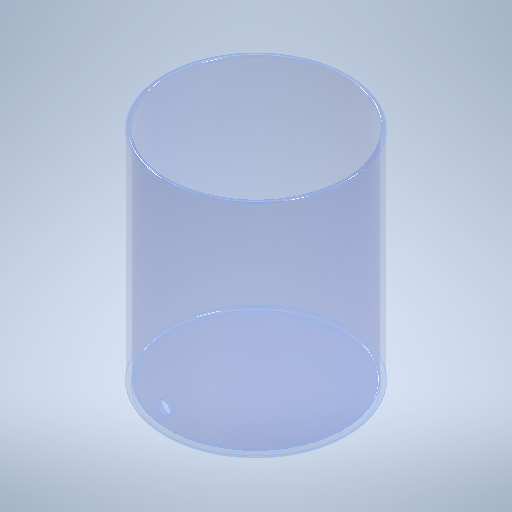
# Autodesk Inventor part: Reservoir
Saved by Autodesk Inventor 2025.2 (Build 292293000, 293)
## iProperties
Created: 2025-05-29
Part Number: Reservoir
Material: Generic
Document SubType Name: Modeling
Designer: Simon
Density: 1 g/cm^3
Appearance: Tropical Blue
Author: Simon
Autodesk Inventor part; units mm, degrees
ref_plane "YZ Plane" through (0, 0, 0) normal (1, 0, 0) x (0, 1, 0)
ref_plane "XZ Plane" through (0, 0, 0) normal (0, 1, 0) x (-1, 0, 0)
ref_plane "XY Plane" through (0, 0, 0) normal (0, 0, 1) x (1, 0, 0)
sketch "Sketch1" plane through (0, 0, 0) normal (0, 1, 0) x (-1, 0, 0)
  circle A0 centre (0, 0) radius 42
  dimension "d0" = 84
  constraints: 1 centre point, 1 coincident
  measures "d0" diameter of A0
extrude "Extrusion1" add sketch "Sketch1" along normal blind 2
sketch "Sketch2" plane through (0, 2, 0) normal (0, 1, 0) x (1, 0, 0)
  circle A0 centre (0, 0) radius 42
  circle A1 centre (0, 0) radius 40
  dimension "d3" = 80
  dimension "d6" = 84
  constraints: 2 centre point, 2 coincident
  measures "d3" diameter of A1
  measures "d6" diameter of A0
extrude "Extrusion2" add sketch "Sketch2" along normal blind 100
fillet "Fillet1" radius 2 1 edges at (42, 0, 0)
fillet "Fillet2" radius 1 2 edges at (-42, 102, 0) (-40, 102, 0)
fillet "Fillet3" radius 1 1 edges at (-40, 2, 0)
sketch "Sketch3" plane through (0, 0, 0) normal (0, 0, 1) x (1, 0, 0)
  line L0 (-42, 2) -> (42, 2) projected
  line L1 (0, 2) -> (0, 12)
  circle A0 centre (0, 12) radius 3
  point P0 (0, 0)
  dimension "d10" = 10
  dimension "d11" = 6
  constraints: 2 end point, 1 centre point, 1 coincident, 1 midpoint, 1 vertical
  measures "d10" distance of L1.start L1.end
  measures "d11" diameter of A0
extrude "Extrusion3" cut sketch "Sketch3" along normal through all
body "Solid1"
